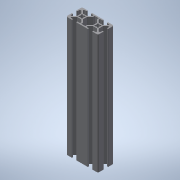
# Autodesk Inventor part: 20-2040_150mm
Saved by Autodesk Inventor 2021 (Build 250183000, 183)
## iProperties
Created: 2014-04-23
Part Number: 20-2040_150mm
Material: Generic
Document SubType Name: Modeling
Designer: Ross Bowman
Density: 1 g/cm^3
Engineer: Ross Bowman
Catalog Web Link: 8020.net
Vendor: 80/20 Inc.
Appearance: Default
Company: 80/20 Inc.
Material: 6105-T5 Aluminum
Author: Ross Bowman
Keywords: 80/20 , 8020 , T-Slot , Extrusion
Autodesk Inventor part; units mm, degrees
ref_plane "YZ Plane" through (0, 0, 0) normal (1, 0, 0) x (0, 1, 0)
ref_plane "XZ Plane" through (0, 0, 0) normal (0, 1, 0) x (-1, 0, 0)
ref_plane "XY Plane" through (0, 0, 0) normal (0, 0, 1) x (1, 0, 0)
sketch "Sketch1" plane through (0, 0, 0) normal (0, 0, 1) x (1, 0, 0)
  arc A0 (-12.1249, -2.3045) -> (-10.804, -1.9351) centre (-11.5684, -1.748) ccw
  line L0 (-12.3045, -2.1249) -> (-12.1249, -2.3045)
  arc A1 (-11.9351, -0.804) -> (-12.3045, -2.1249) centre (-11.748, -1.5684) ccw
  arc A2 (-11.9351, 0.804) -> (-11.9351, -0.804) centre (-10, 0) ccw
  arc A3 (-12.3045, 2.1249) -> (-11.9351, 0.804) centre (-11.748, 1.5684) ccw
  line L1 (-12.1249, 2.3045) -> (-12.3045, 2.1249)
  arc A4 (-10.804, 1.9351) -> (-12.1249, 2.3045) centre (-11.5684, 1.748) ccw
  arc A5 (-9.196, 1.9351) -> (-10.804, 1.9351) centre (-10, 0) ccw
  arc A6 (-7.8751, 2.3045) -> (-9.196, 1.9351) centre (-8.4316, 1.748) ccw
  line L2 (-7.6955, 2.1249) -> (-7.8751, 2.3045)
  arc A7 (-8.0649, 0.804) -> (-7.6955, 2.1249) centre (-8.252, 1.5684) ccw
  arc A8 (-8.0649, -0.804) -> (-8.0649, 0.804) centre (-10, 0) ccw
  arc A9 (-7.6955, -2.1249) -> (-8.0649, -0.804) centre (-8.252, -1.5684) ccw
  line L3 (-7.8751, -2.3045) -> (-7.6955, -2.1249)
  arc A10 (-9.196, -1.9351) -> (-7.8751, -2.3045) centre (-8.4316, -1.748) ccw
  arc A11 (-10.804, -1.9351) -> (-9.196, -1.9351) centre (-10, 0) ccw
  arc A12 (-2.505, -7.992) -> (-1.997, -8.5) centre (-1.997, -7.992) ccw
  line L4 (-2.505, -6.6448) -> (-2.505, -7.992)
  arc A13 (-2.505, -6.6448) -> (-2.6538, -6.2856) centre (-3.013, -6.6448) ccw
  line L5 (-6.1962, -2.7431) -> (-2.6538, -6.2856)
  arc A14 (-6.345, -2.3839) -> (-6.1962, -2.7431) centre (-5.837, -2.3839) ccw
  line L6 (-6.345, 2.3839) -> (-6.345, -2.3839)
  arc A15 (-6.1962, 2.7431) -> (-6.345, 2.3839) centre (-5.837, 2.3839) ccw
  line L7 (-2.6538, 6.2856) -> (-6.1962, 2.7431)
  arc A16 (-2.6538, 6.2856) -> (-2.505, 6.6448) centre (-3.013, 6.6448) ccw
  line L8 (-2.505, 7.992) -> (-2.505, 6.6448)
  arc A17 (-1.997, 8.5) -> (-2.505, 7.992) centre (-1.997, 7.992) ccw
  line L9 (1.997, 8.5) -> (-1.997, 8.5)
  arc A18 (2.505, 7.992) -> (1.997, 8.5) centre (1.997, 7.992) ccw
  line L10 (2.505, 6.6448) -> (2.505, 7.992)
  arc A19 (2.505, 6.6448) -> (2.6538, 6.2856) centre (3.013, 6.6448) ccw
  line L11 (6.1962, 2.7431) -> (2.6538, 6.2856)
  arc A20 (6.345, 2.3839) -> (6.1962, 2.7431) centre (5.837, 2.3839) ccw
  line L12 (6.345, -2.3839) -> (6.345, 2.3839)
  arc A21 (6.1962, -2.7431) -> (6.345, -2.3839) centre (5.837, -2.3839) ccw
  line L13 (2.6538, -6.2856) -> (6.1962, -2.7431)
  arc A22 (2.6538, -6.2856) -> (2.505, -6.6448) centre (3.013, -6.6448) ccw
  line L14 (2.505, -7.992) -> (2.505, -6.6448)
  arc A23 (1.997, -8.5) -> (2.505, -7.992) centre (1.997, -7.992) ccw
  line L15 (-1.997, -8.5) -> (1.997, -8.5)
  arc A24 (7.8751, -2.3045) -> (9.196, -1.9351) centre (8.4316, -1.748) ccw
  line L16 (7.6955, -2.1249) -> (7.8751, -2.3045)
  arc A25 (8.0649, -0.804) -> (7.6955, -2.1249) centre (8.252, -1.5684) ccw
  arc A26 (8.0649, 0.804) -> (8.0649, -0.804) centre (10, 0) ccw
  arc A27 (7.6955, 2.1249) -> (8.0649, 0.804) centre (8.252, 1.5684) ccw
  line L17 (7.8751, 2.3045) -> (7.6955, 2.1249)
  arc A28 (9.196, 1.9351) -> (7.8751, 2.3045) centre (8.4316, 1.748) ccw
  arc A29 (10.804, 1.9351) -> (9.196, 1.9351) centre (10, 0) ccw
  arc A30 (12.1249, 2.3045) -> (10.804, 1.9351) centre (11.5684, 1.748) ccw
  line L18 (12.3045, 2.1249) -> (12.1249, 2.3045)
  arc A31 (11.9351, 0.804) -> (12.3045, 2.1249) centre (11.748, 1.5684) ccw
  arc A32 (11.9351, -0.804) -> (11.9351, 0.804) centre (10, 0) ccw
  arc A33 (12.3045, -2.1249) -> (11.9351, -0.804) centre (11.748, -1.5684) ccw
  line L19 (12.1249, -2.3045) -> (12.3045, -2.1249)
  arc A34 (10.804, -1.9351) -> (12.1249, -2.3045) centre (11.5684, -1.748) ccw
  arc A35 (9.196, -1.9351) -> (10.804, -1.9351) centre (10, 0) ccw
  arc A36 (-12.3839, -3.655) -> (-12.7431, -3.8038) centre (-12.3839, -4.163) ccw
  line L20 (-12.3839, -3.655) -> (-7.6161, -3.655)
  arc A37 (-7.2569, -3.8038) -> (-7.6161, -3.655) centre (-7.6161, -4.163) ccw
  line L21 (-7.2569, -3.8038) -> (-4.1538, -6.9069)
  arc A38 (-4.005, -7.2661) -> (-4.1538, -6.9069) centre (-4.513, -7.2661) ccw
  line L22 (-4.005, -7.2661) -> (-4.005, -7.992)
  arc A39 (-4.513, -8.5) -> (-4.005, -7.992) centre (-4.513, -7.992) ccw
  line L23 (-4.513, -8.5) -> (-6.862, -8.5)
  arc A40 (-6.862, -8.5) -> (-7.37, -9.008) centre (-6.862, -9.008) ccw
  line L24 (-7.37, -9.008) -> (-7.37, -9.492)
  arc A41 (-7.37, -9.492) -> (-6.862, -10) centre (-6.862, -9.492) ccw
  line L25 (-6.862, -10) -> (6.862, -10)
  arc A42 (6.862, -10) -> (7.37, -9.492) centre (6.862, -9.492) ccw
  line L26 (7.37, -9.492) -> (7.37, -9.008)
  arc A43 (7.37, -9.008) -> (6.862, -8.5) centre (6.862, -9.008) ccw
  line L27 (6.862, -8.5) -> (4.513, -8.5)
  arc A44 (4.005, -7.992) -> (4.513, -8.5) centre (4.513, -7.992) ccw
  line L28 (4.005, -7.992) -> (4.005, -7.2661)
  arc A45 (4.1538, -6.9069) -> (4.005, -7.2661) centre (4.513, -7.2661) ccw
  line L29 (4.1538, -6.9069) -> (7.2569, -3.8038)
  arc A46 (7.6161, -3.655) -> (7.2569, -3.8038) centre (7.6161, -4.163) ccw
  line L30 (7.6161, -3.655) -> (12.3839, -3.655)
  arc A47 (12.7431, -3.8038) -> (12.3839, -3.655) centre (12.3839, -4.163) ccw
  line L31 (12.7431, -3.8038) -> (15.8462, -6.9069)
  arc A48 (15.995, -7.2661) -> (15.8462, -6.9069) centre (15.487, -7.2661) ccw
  line L32 (15.995, -7.2661) -> (15.995, -7.992)
  arc A49 (15.487, -8.5) -> (15.995, -7.992) centre (15.487, -7.992) ccw
  line L33 (15.487, -8.5) -> (13.138, -8.5)
  arc A50 (13.138, -8.5) -> (12.63, -9.008) centre (13.138, -9.008) ccw
  line L34 (12.63, -9.008) -> (12.63, -9.492)
  arc A51 (12.63, -9.492) -> (13.138, -10) centre (13.138, -9.492) ccw
  line L35 (13.138, -10) -> (18.5, -10)
  arc A52 (18.5, -10) -> (20, -8.5) centre (18.5, -8.5) ccw
  line L36 (20, -8.5) -> (20, -3.138)
  arc A53 (20, -3.138) -> (19.492, -2.63) centre (19.492, -3.138) ccw
  line L37 (19.492, -2.63) -> (19.008, -2.63)
  arc A54 (19.008, -2.63) -> (18.5, -3.138) centre (19.008, -3.138) ccw
  line L38 (18.5, -3.138) -> (18.5, -5.487)
  arc A55 (17.992, -5.995) -> (18.5, -5.487) centre (17.992, -5.487) ccw
  line L39 (17.992, -5.995) -> (17.2661, -5.995)
  arc A56 (16.9069, -5.8462) -> (17.2661, -5.995) centre (17.2661, -5.487) ccw
  line L40 (16.9069, -5.8462) -> (13.8038, -2.7431)
  arc A57 (13.655, -2.3839) -> (13.8038, -2.7431) centre (14.163, -2.3839) ccw
  line L41 (13.655, -2.3839) -> (13.655, 2.3839)
  arc A58 (13.8038, 2.7431) -> (13.655, 2.3839) centre (14.163, 2.3839) ccw
  line L42 (13.8038, 2.7431) -> (16.9069, 5.8462)
  arc A59 (17.2661, 5.995) -> (16.9069, 5.8462) centre (17.2661, 5.487) ccw
  line L43 (17.2661, 5.995) -> (17.992, 5.995)
  arc A60 (18.5, 5.487) -> (17.992, 5.995) centre (17.992, 5.487) ccw
  line L44 (18.5, 5.487) -> (18.5, 3.138)
  arc A61 (18.5, 3.138) -> (19.008, 2.63) centre (19.008, 3.138) ccw
  line L45 (19.008, 2.63) -> (19.492, 2.63)
  arc A62 (19.492, 2.63) -> (20, 3.138) centre (19.492, 3.138) ccw
  line L46 (20, 3.138) -> (20, 8.5)
  arc A63 (20, 8.5) -> (18.5, 10) centre (18.5, 8.5) ccw
  line L47 (18.5, 10) -> (13.138, 10)
  arc A64 (13.138, 10) -> (12.63, 9.492) centre (13.138, 9.492) ccw
  line L48 (12.63, 9.492) -> (12.63, 9.008)
  arc A65 (12.63, 9.008) -> (13.138, 8.5) centre (13.138, 9.008) ccw
  line L49 (13.138, 8.5) -> (15.487, 8.5)
  arc A66 (15.995, 7.992) -> (15.487, 8.5) centre (15.487, 7.992) ccw
  line L50 (15.995, 7.992) -> (15.995, 7.2661)
  arc A67 (15.8462, 6.9069) -> (15.995, 7.2661) centre (15.487, 7.2661) ccw
  line L51 (15.8462, 6.9069) -> (12.7431, 3.8038)
  arc A68 (12.3839, 3.655) -> (12.7431, 3.8038) centre (12.3839, 4.163) ccw
  line L52 (12.3839, 3.655) -> (7.6161, 3.655)
  arc A69 (7.2569, 3.8038) -> (7.6161, 3.655) centre (7.6161, 4.163) ccw
  line L53 (7.2569, 3.8038) -> (4.1538, 6.9069)
  arc A70 (4.005, 7.2661) -> (4.1538, 6.9069) centre (4.513, 7.2661) ccw
  line L54 (4.005, 7.2661) -> (4.005, 7.992)
  arc A71 (4.513, 8.5) -> (4.005, 7.992) centre (4.513, 7.992) ccw
  line L55 (4.513, 8.5) -> (6.862, 8.5)
  arc A72 (6.862, 8.5) -> (7.37, 9.008) centre (6.862, 9.008) ccw
  line L56 (7.37, 9.008) -> (7.37, 9.492)
  arc A73 (7.37, 9.492) -> (6.862, 10) centre (6.862, 9.492) ccw
  line L57 (6.862, 10) -> (-6.862, 10)
  arc A74 (-6.862, 10) -> (-7.37, 9.492) centre (-6.862, 9.492) ccw
  line L58 (-7.37, 9.492) -> (-7.37, 9.008)
  arc A75 (-7.37, 9.008) -> (-6.862, 8.5) centre (-6.862, 9.008) ccw
  line L59 (-6.862, 8.5) -> (-4.513, 8.5)
  arc A76 (-4.005, 7.992) -> (-4.513, 8.5) centre (-4.513, 7.992) ccw
  line L60 (-4.005, 7.992) -> (-4.005, 7.2661)
  arc A77 (-4.1538, 6.9069) -> (-4.005, 7.2661) centre (-4.513, 7.2661) ccw
  line L61 (-4.1538, 6.9069) -> (-7.2569, 3.8038)
  arc A78 (-7.6161, 3.655) -> (-7.2569, 3.8038) centre (-7.6161, 4.163) ccw
  line L62 (-7.6161, 3.655) -> (-12.3839, 3.655)
  arc A79 (-12.7431, 3.8038) -> (-12.3839, 3.655) centre (-12.3839, 4.163) ccw
  line L63 (-12.7431, 3.8038) -> (-15.8462, 6.9069)
  arc A80 (-15.995, 7.2661) -> (-15.8462, 6.9069) centre (-15.487, 7.2661) ccw
  line L64 (-15.995, 7.2661) -> (-15.995, 7.992)
  arc A81 (-15.487, 8.5) -> (-15.995, 7.992) centre (-15.487, 7.992) ccw
  line L65 (-15.487, 8.5) -> (-13.138, 8.5)
  arc A82 (-13.138, 8.5) -> (-12.63, 9.008) centre (-13.138, 9.008) ccw
  line L66 (-12.63, 9.008) -> (-12.63, 9.492)
  arc A83 (-12.63, 9.492) -> (-13.138, 10) centre (-13.138, 9.492) ccw
  line L67 (-13.138, 10) -> (-18.5, 10)
  arc A84 (-18.5, 10) -> (-20, 8.5) centre (-18.5, 8.5) ccw
  line L68 (-20, 8.5) -> (-20, 3.138)
  arc A85 (-20, 3.138) -> (-19.492, 2.63) centre (-19.492, 3.138) ccw
  line L69 (-19.492, 2.63) -> (-19.008, 2.63)
  arc A86 (-19.008, 2.63) -> (-18.5, 3.138) centre (-19.008, 3.138) ccw
  line L70 (-18.5, 3.138) -> (-18.5, 5.487)
  arc A87 (-17.992, 5.995) -> (-18.5, 5.487) centre (-17.992, 5.487) ccw
  line L71 (-17.992, 5.995) -> (-17.2661, 5.995)
  arc A88 (-16.9069, 5.8462) -> (-17.2661, 5.995) centre (-17.2661, 5.487) ccw
  line L72 (-16.9069, 5.8462) -> (-13.8038, 2.7431)
  arc A89 (-13.655, 2.3839) -> (-13.8038, 2.7431) centre (-14.163, 2.3839) ccw
  line L73 (-13.655, 2.3839) -> (-13.655, -2.3839)
  arc A90 (-13.8038, -2.7431) -> (-13.655, -2.3839) centre (-14.163, -2.3839) ccw
  line L74 (-13.8038, -2.7431) -> (-16.9069, -5.8462)
  arc A91 (-17.2661, -5.995) -> (-16.9069, -5.8462) centre (-17.2661, -5.487) ccw
  line L75 (-17.2661, -5.995) -> (-17.992, -5.995)
  arc A92 (-18.5, -5.487) -> (-17.992, -5.995) centre (-17.992, -5.487) ccw
  line L76 (-18.5, -5.487) -> (-18.5, -3.138)
  arc A93 (-18.5, -3.138) -> (-19.008, -2.63) centre (-19.008, -3.138) ccw
  line L77 (-19.008, -2.63) -> (-19.492, -2.63)
  arc A94 (-19.492, -2.63) -> (-20, -3.138) centre (-19.492, -3.138) ccw
  line L78 (-20, -3.138) -> (-20, -8.5)
  arc A95 (-20, -8.5) -> (-18.5, -10) centre (-18.5, -8.5) ccw
  line L79 (-18.5, -10) -> (-13.138, -10)
  arc A96 (-13.138, -10) -> (-12.63, -9.492) centre (-13.138, -9.492) ccw
  line L80 (-12.63, -9.492) -> (-12.63, -9.008)
  arc A97 (-12.63, -9.008) -> (-13.138, -8.5) centre (-13.138, -9.008) ccw
  line L81 (-13.138, -8.5) -> (-15.487, -8.5)
  arc A98 (-15.995, -7.992) -> (-15.487, -8.5) centre (-15.487, -7.992) ccw
  line L82 (-15.995, -7.992) -> (-15.995, -7.2661)
  arc A99 (-15.8462, -6.9069) -> (-15.995, -7.2661) centre (-15.487, -7.2661) ccw
  line L83 (-15.8462, -6.9069) -> (-12.7431, -3.8038)
  point P0 (0, 0)
  constraints: 200 point on circle, 168 end point, 100 centre point
extrude "Extrusion1" add sketch "Sketch1" against normal blind 100
move faces "Move1" translate (0, 0, 50) faces at (-0.6657, -9.5, 0)
body "Solid1"
